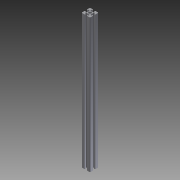
# Autodesk Inventor part: Alu-Profil Nut 10 45x45 710
Saved by Autodesk Inventor 2012 SP1 (Build 160190100, 190)
## iProperties
Created: 2013-01-29
Part Number: Alu-Profil Nut 10 45x45 710
Material: Default
Document SubType Name: Modeling
Designer: vogel
Density: 1 g/cm^3
Author: vogel
Autodesk Inventor part; units mm, degrees
ref_plane "YZ Plane" through (0, 0, 0) normal (1, 0, 0) x (0, 1, 0)
ref_plane "XZ Plane" through (0, 0, 0) normal (0, 1, 0) x (-1, 0, 0)
ref_plane "XY Plane" through (0, 0, 0) normal (0, 0, 1) x (1, 0, 0)
sketch "Skizze1" plane through (0, 0, 0) normal (0, 0, 1) x (1, 0, 0)
  line L0 (-19.5, 22.5) -> (19.5, 22.5)
  line L1 (22.5, 19.5) -> (22.5, -19.5)
  line L2 (19.5, -22.5) -> (-19.5, -22.5)
  line L3 (-22.5, -19.5) -> (-22.5, 19.5)
  circle A0 centre (0, 0) radius 5
  line L4 (-32.3698, 0) -> (32.3698, 0) projected
  line L5 (0, -32.3698) -> (0, 32.3698) projected
  arc A1 (22.5, 19.5) -> (19.5, 22.5) centre (19.5, 19.5) ccw
  arc A2 (-19.5, 22.5) -> (-22.5, 19.5) centre (-19.5, 19.5) ccw
  arc A3 (-22.5, -19.5) -> (-19.5, -22.5) centre (-19.5, -19.5) ccw
  arc A4 (19.5, -22.5) -> (22.5, -19.5) centre (19.5, -19.5) ccw
  point P0 (-22.5, 22.5)
  point P1 (22.5, 22.5)
  point P2 (-22.5, -22.5)
  dimension "d0" = 45
  dimension "d1" = 45
  dimension "d2" = 10
  dimension "d3" = 3
  constraints: 8 end point, 8 point on circle, 8 tangent, 6 point on line, 5 centre point, 3 equal radius, 2 parallel, 1 coincident, 1 horizontal, 1 perpendicular, 2 other
  measures "d0" distance of point (-22.5, -22.5) point (-22.5, 22.5)
  measures "d1" distance of point (-22.5, 22.5) point (22.5, 22.5)
  measures "d2" diameter of A0
  measures "d3" radius of A1
extrude "Extrusion1" add sketch "Skizze1" along normal blind 710 contours L0 L5 A0 L4 L3 A2 | L0 A1 L1 L4 A0 L5 | L4 A0 L5 L2 A3 L3 | L4 L1 A4 L2 L5 A0
sketch "Skizze2" plane through (0, 0, 0) normal (0, 0, -1) x (-1, 0, 0)
  line L0 (19.5, -22.5) -> (-19.5, -22.5) projected
  line L1 (31.5, 0) -> (-31.5, 0) projected
  line L2 (0, -31.5) -> (0, 31.5) projected
  line L3 (-6, -22.5) -> (-6, -21)
  line L4 (-6, -21) -> (-5, -21)
  line L5 (-5, -21) -> (-5, -16.5)
  line L6 (-5, -16.5) -> (-10, -16.5)
  line L7 (-10, -16.5) -> (-10, -13)
  line L8 (-10, -13) -> (-7, -10)
  line L9 (-7, -10) -> (7, -10)
  line L10 (7, -10) -> (10, -13)
  line L11 (10, -13) -> (10, -16.5)
  line L12 (10, -16.5) -> (5, -16.5)
  line L13 (5, -16.5) -> (5, -21)
  line L14 (5, -21) -> (6, -21)
  line L15 (6, -21) -> (6, -22.5)
  dimension "d6" = 10
  dimension "d7" = 20
  dimension "d8" = 12
  dimension "d9" = 1.5
  dimension "d10" = 12.5
  dimension "d11" = 135
  dimension "d12" = 6
  dimension "d13" = 3.5
  constraints: 26 end point, 8 parallel, 3 collinear, 2 perpendicular, 2 point on line, 4 other
  measures "d6" distance between parallel lines of L5 L13
  measures "d7" distance between parallel lines of L11 L7
  measures "d8" distance between parallel lines of L3 L15
  measures "d9" distance between parallel lines of L14 L0
  measures "d10" distance between parallel lines of L9 L0
  measures "d11" angle of L9 L10
  measures "d12" distance between parallel lines of L0 L12
  measures "d13" distance of L10.end L11.end
extrude "Extrusion2" cut sketch "Skizze2" against normal through all
pattern_circular "Runde Anordnung1" count 4 over 360 about axis through (0, 0, 0) along (0, 0, 1) of "Extrusion2"
sketch "Skizze3" plane through (0, 0, 0) normal (0, 0, -1) x (-1, 0, 0)
  circle A0 centre (0, 0) radius 5 projected
  line L0 (31.5, 0) -> (-31.5, 0) projected
  line L1 (0, -31.5) -> (0, 31.5) projected
  line L2 (-1.5708, 7.8443) -> (-0.9817, 4.9027)
  line L3 (1.5708, 7.8443) -> (0.9817, 4.9027)
  arc A1 (1.5708, 7.8443) -> (-1.5708, 7.8443) centre (0, 0) ccw
  dimension "d20" = 1.9635
  dimension "d21" = 3.1416
  dimension "d22" = 8
  constraints: 4 end point, 4 point on circle, 1 centre point, 1 coincident, 1 other
  measures "d20" distance of L3.end L2.end
  measures "d21" distance of L3.start L2.start
  measures "d22" radius of A1
extrude "Extrusion3" cut sketch "Skizze3" against normal through all contours A0 L1 A1 L3 | A0 L2 A1 L1
pattern_circular "Runde Anordnung2" count 8 over 360 about axis through (0, 0, 0) along (0, 0, 1) of "Extrusion3"
